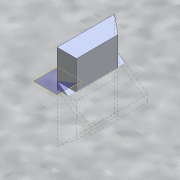
# Autodesk Inventor part: ReaderV2
Saved by Autodesk Inventor 2016 (Build 200138000, 138)
## iProperties
Created: 2016-01-17
Part Number: ReaderV2
Material: Generic
Document SubType Name: Modeling
Designer: Drew
Density: 1 g/cm^3
Appearance: Default
Author: Drew
Autodesk Inventor part; units mm, degrees
ref_plane "YZ Plane" through (0, 0, 0) normal (1, 0, 0) x (0, 1, 0)
ref_plane "XZ Plane" through (0, 0, 0) normal (0, 1, 0) x (-1, 0, 0)
sketch "Body Base Sketch" plane through (0, 0, 0) normal (1, 0, 0) x (0, 1, 0)
  line L0 (96.9938, 25.4) -> (20.7938, 25.4)
  line L1 (20.7938, 25.4) -> (20.7938, -25.4)
  line L2 (20.7938, -25.4) -> (96.9938, -25.4)
  line L3 (96.9938, -25.4) -> (96.9938, 25.4)
  line L4 (96.9938, 25.4) -> (20.7938, -25.4)
  line L5 (-19.3988, 0) -> (116.3926, 0)
  point P0 (0, 0)
  point P1 (58.8938, 0)
  dimension "d0" = 76.2
  dimension "d1" = 50.8
  constraints: 12 end point, 2 parallel, 1 horizontal, 1 midpoint, 1 perpendicular, 1 point on line
  measures "d0" distance of L2.end L1.end
  measures "d1" distance of L0.end L1.end
extrude "Body Extrusion" add sketch "Body Base Sketch" along normal blind 10.16
ref_plane "Left Side Plane" through (0, 96.9938, 25.4) normal (0, 0, 1) x (1, 0, 0)
ref_plane "Right Side Plane" through (0, 96.9938, -25.4) normal (0, 0, 1) x (1, 0, 0)
draft "Body Draft" angle 35 pull direction (1, 0, 0) fixed plane through (0, 71.5938, -8.4667) normal (-1, 0, 0) faces at (6.7733, 71.5938, 25.4) (6.7733, 96.9938, -8.4667) (3.3867, 46.1938, -25.4) (6.7733, 20.7938, 8.4667)
sketch "RFID Plate Sketch" plane through (0, 0, 0) normal (0, 0, 1) x (1, 0, 0)
  line L0 (0, 70.9939) -> (29.4248, 50.3904)
  line L1 (0, 64.6439) -> (29.4248, 44.0404)
  line L2 (0, 70.9939) -> (0, 64.6439)
  line L3 (29.4248, 50.3904) -> (29.4248, 44.0404)
  line L4 (0, 96.9938) -> (10.16, 89.8797) projected
  line L5 (0, 96.9938) -> (0, 20.7938) projected
  point P0 (0, 0)
  dimension "d9" = 6.35
  constraints: 8 end point, 2 parallel, 1 collinear, 1 vertical, 1 vertical alignment
  measures "d9" distance of L0.end L1.end
extrude "RFID Plane Extrusion" add sketch "RFID Plate Sketch" against normal up to surface (50.8 mm away) from surface at 25.4
ref_plane "RFID Top Hortizontal Plane" through (0, 70.9939, 25.4) normal (0, -1, 0) x (1, 0, 0)
body "Solid1"
